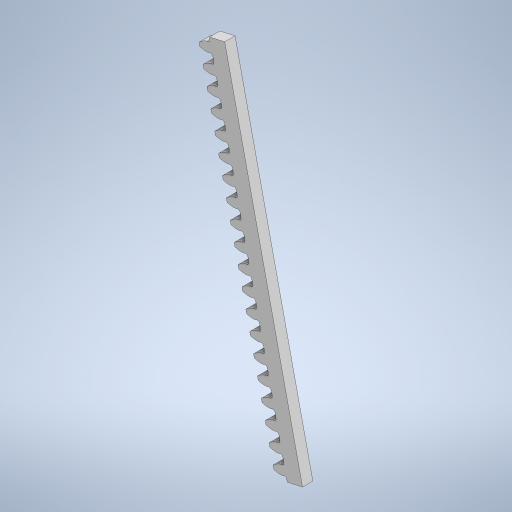
# Autodesk Inventor part: 零件3
Saved by Autodesk Inventor 2024 (Build 280153000, 153)
## iProperties
Created: 2024-04-21
Part Number: 零件3
Material: 一般
Document SubType Name: Modeling
Designer: rumse
Density: 1 g/cm^3
Appearance: 預設
Author: rumse
Autodesk Inventor part; units mm, degrees
ref_plane "YZ Plane" through (0, 0, 0) normal (1, 0, 0) x (0, 1, 0)
ref_plane "XZ Plane" through (0, 0, 0) normal (0, 1, 0) x (-1, 0, 0)
ref_plane "XY Plane" through (0, 0, 0) normal (0, 0, 1) x (1, 0, 0)
sketch "草圖1" plane through (0, 0, 0) normal (0, 0, 1) x (1, 0, 0)
  arc A0 (-1.4025, 1.1427) -> (-1.6393, 1.2572) centre (-1.5806, 1.0765) ccw
  line L0 (-1.6393, 1.2572) -> (-1.77, 1.2147)
  arc A1 (-1.8256, 2.0877) -> (-1.6604, 2.2924) centre (-1.8498, 2.2762) ccw
  line L1 (-1.9619, 2.0703) -> (-1.8256, 2.0877)
  spline S0 degree 4 poles (-2.7034, 1.6326) (-2.669, 1.6638) (-2.6174, 1.7085) (-2.5492, 1.7636) (-2.4658, 1.825) (-2.402, 1.8686) (-2.3415, 1.9069) (-2.2847, 1.9402) (-2.2318, 1.9688) (-2.1831, 1.9929) (-2.1387, 2.013) (-2.099, 2.0294) (-2.0642, 2.0424) (-2.0343, 2.0523) (-2.0097, 2.0596) (-1.9862, 2.0657) (-1.9721, 2.0687) (-1.9637, 2.0701) (-1.9619, 2.0703) knots 0.046846 0.046846 0.046846 0.046846 0.046846 0.199152 0.275088 0.348442 0.419118 0.487011 0.551999 0.613947 0.672693 0.728051 0.779794 0.827641 0.871232 0.910072 0.943417 1 1 1 1 1
  arc A2 (-2.7034, 1.6326) -> (-2.6274, 1.2937) centre (2.6985, 2.6667) ccw
  spline S1 degree 4 poles (-1.77, 1.2147) (-1.7717, 1.2142) (-1.7799, 1.2118) (-1.7939, 1.2086) (-1.8178, 1.204) (-1.8431, 1.2001) (-1.8744, 1.1963) (-1.9114, 1.1932) (-1.9543, 1.191) (-2.003, 1.1902) (-2.0573, 1.1912) (-2.1174, 1.1945) (-2.183, 1.2003) (-2.254, 1.2091) (-2.3303, 1.2213) (-2.432, 1.2411) (-2.5172, 1.2618) (-2.583, 1.2802) (-2.6274, 1.2937) knots 0 0 0 0 0 0.056583 0.089928 0.128768 0.172359 0.220206 0.271949 0.327307 0.386053 0.448001 0.512989 0.580882 0.651558 0.724912 0.800848 0.953154 0.953154 0.953154 0.953154 0.953154
  arc A3 (-1.4025, 1.1427) -> (-1.3315, 0.9638) centre (2.6985, 2.6667) ccw
  arc A4 (-1.6727, 2.4846) -> (-1.6604, 2.2924) centre (2.6985, 2.6667) ccw
  arc A5 (-1.3166, 0.8839) -> (-1.3315, 0.9638) centre (-1.5065, 0.8898) ccw
  arc A6 (-1.6727, 2.4846) -> (-1.6934, 2.5631) centre (-1.8625, 2.4767) ccw
  line L2 (-1.3166, 0.8839) -> (0.147, 1.2123)
  line L3 (0.147, 1.2123) -> (-0.2297, 2.8915)
  line L4 (-0.2297, 2.8915) -> (-1.6934, 2.5631)
  point P0 (0, 0)
  constraints: 14 centre point, 14 point on circle, 10 end point, 8 other
extrude "擠出1" add sketch "草圖1" along normal blind 1
pattern_linear "矩形陣列1" count 20 spacing 1.721 along (-0.218927, 0.9757413, 0) of "擠出1"
